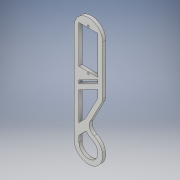
# Autodesk Inventor part: Pata - Brazo
Saved by Autodesk Inventor 2019 (Build 230136000, 136)
## iProperties
Created: 2020-02-12
Part Number: Pata - Brazo
Material: Generic
Document SubType Name: Modeling
Designer: jacqu
Density: 1 g/cm^3
Appearance: Default
Mass: 11.5957 g
Surface Area: 94.6447 cm^2
Volume: 11.5957 cm^3
Author: jacqu
Autodesk Inventor part; units mm, degrees
ref_plane "YZ Plane" through (0, 0, 0) normal (1, 0, 0) x (0, 1, 0)
ref_plane "XZ Plane" through (0, 0, 0) normal (0, 1, 0) x (-1, 0, 0)
ref_plane "XY Plane" through (0, 0, 0) normal (0, 0, 1) x (1, 0, 0)
sketch "Sketch1" plane through (0, 0, 0) normal (0, 0, 1) x (1, 0, 0)
  arc A0 (15, 0) -> (-15, 0) centre (0, 0) ccw
  line L0 (-15, 0) -> (-15, -104)
  line L1 (15, 0) -> (15, -52)
  arc A1 (14.2508, -55.0541) -> (15, -52) centre (8.4, -52) ccw
  arc A2 (-15, -104) -> (-5.2894, -118.0365) centre (0, -104) ccw
  arc A3 (-5.2894, -118.0365) -> (14.9722, -104.9126) centre (0, -104) ccw
  arc A4 (14.9722, -104.9126) -> (5.7487, -90.1453) centre (0, -104) ccw
  arc A5 (1.7228, -79.0541) -> (5.7487, -90.1453) centre (8.8147, -82.7561) ccw
  line L2 (1.7228, -79.0541) -> (14.2508, -55.0541)
  line L3 (-10, 5.5) -> (10, 5.5)
  line L4 (10, 5.5) -> (10, -34.5)
  line L5 (10, -34.5) -> (-10, -34.5)
  line L6 (-10, -34.5) -> (-10, 5.5)
  dimension "d3" = 15
  dimension "d5" = 52
  dimension "d6" = 15
  dimension "d7" = 15
  dimension "d8" = 8
  dimension "d10" = 6.6
  dimension "d11" = 24
  dimension "d17" = 20
  dimension "d18" = 40
  dimension "d19" = 10
  dimension "d20" = 104
  dimension "d30" = 5.5
  constraints: 14 end point, 13 point on circle, 8 tangent, 6 centre point, 3 parallel, 1 coincident, 1 concentric, 1 horizontal, 1 perpendicular, 1 vertical alignment
  measures "d3" radius of A0
  measures "d5" distance of L1.start L1.end
  measures "d6" radius of A2
  measures "d7" radius of A4
  measures "d8" radius of A5
  measures "d10" radius of A1
  measures "d11" vertical distance of L2.start L2.end
  measures "d17" distance of L3.start L3.end
  measures "d18" distance of L3.end L4.end
  measures "d19" distance from line of L6 point (0, 0)
  measures "d20" distance of L0.start L0.end
  measures "d30" distance from line of point (0, 0) L3
extrude "Extrusion1" add sketch "Sketch1" along normal blind 3.3
sketch "Sketch2" plane through (0, 0, 3.3) normal (0, 0, 1) x (1, 0, 0)
  line L0 (-10, 5.5) -> (10, 5.5) projected
  line L1 (10, -34.5) -> (-10, -34.5) projected
  circle A0 centre (0, 7.25) radius 1
  circle A1 centre (0, -36.25) radius 1
  point P0 (0, 0)
  dimension "d31" = 2
  dimension "d32" = 2
  dimension "d34" = 1.75
  dimension "d36" = 1.75
  constraints: 2 centre point, 2 vertical alignment
  measures "d31" diameter of A0
  measures "d32" diameter of A1
  measures "d34" distance from line of L0 A0.centre
  measures "d36" distance from line of L1 A1.centre
extrude "Extrusion2" cut sketch "Sketch2" against normal blind 3.3
sketch "Sketch3" plane through (0, 0, 3.3) normal (0, 0, 1) x (1, 0, 0)
  line L0 (-15, 0) -> (-15, -104) projected
  circle A0 centre (0, 7.25) radius 1 projected
  circle A1 centre (0, -36.25) radius 1 projected
  line L1 (10, 5.5) -> (10, -34.5) projected
  line L2 (10, -34.5) -> (-10, -34.5) projected
  line L3 (-10, -34.5) -> (-10, 5.5) projected
  line L4 (-10, 5.5) -> (10, 5.5) projected
  line L5 (-15, 0) -> (-15, -104) projected
  arc A2 (-15, -104) -> (5.7487, -90.1453) centre (0, -104) ccw projected
  arc A3 (1.7228, -79.0541) -> (5.7487, -90.1453) centre (8.8147, -82.7561) ccw projected
  line L6 (1.7228, -79.0541) -> (14.2508, -55.0541) projected
  arc A4 (14.2508, -55.0541) -> (15, -52) centre (8.4, -52) ccw projected
  line L7 (15, -52) -> (15, 0) projected
  arc A5 (15, 0) -> (-15, 0) centre (0, 0) ccw projected
  line L8 (-10, -86) -> (-10, -56)
  line L9 (10, -45.5723) -> (10, -53.5723)
  line L10 (10, -53.5723) -> (-3.3016, -79.0541)
  line L11 (-3.3016, -79.0541) -> (-10, -86)
  line L12 (1.7228, -79.0541) -> (14.2508, -55.0541) projected
  line L13 (-10, -97.5245) -> (-10, -104)
  arc A6 (-10, -104) -> (3.8325, -94.7635) centre (0, -104) ccw
  arc A7 (-15, -104) -> (5.7487, -90.1453) centre (0, -104) ccw projected
  arc A8 (-2.2846, -89.5242) -> (3.8325, -94.7635) centre (8.8147, -82.7561) ccw
  arc A9 (1.7228, -79.0541) -> (5.7487, -90.1453) centre (8.8147, -82.7561) ccw projected
  line L14 (-2.2846, -89.5242) -> (-10, -97.5245)
  line L15 (-10, -56) -> (10, -45.5723)
  line L16 (-10, -50.3612) -> (10, -39.9336)
  line L17 (10, -39.9336) -> (10, -36.5503)
  line L18 (10, -36.5503) -> (-10, -46.9779)
  line L19 (-10, -46.9779) -> (-10, -50.3612)
  point P0 (14.81, -53.5723)
  dimension "d45" = 5
  dimension "d46" = 5
  dimension "d48" = 8
  dimension "d49" = 18
  dimension "d52" = 5
  dimension "d54" = 3
  dimension "d56" = 30
  dimension "d57" = 8
  constraints: 22 end point, 6 parallel, 5 point on circle, 3 vertical, 3 vertical alignment, 2 centre point, 2 concentric, 2 horizontal alignment, 2 tangent
  measures "d45" distance between parallel lines of L8 L0
  measures "d46" distance between parallel lines of L7 L9
  measures "d48" distance from line of L8.start L14
  measures "d49" vertical distance of L0.end L8.start
  measures "d52" distance between parallel lines of L15 L16
  measures "d54" distance between parallel lines of L16 L18
  measures "d56" distance of L8.start L8.end
  measures "d57" distance of L9.start L9.end
extrude "Extrusion5" cut sketch "Sketch3" against normal blind 10 contours L8 L15 L9 L10 L11 | L14 A8 A6 L13 | L19 L18 L17 L16
equation "\"d3\" = radio_muslo"
equation "\"d6\" = radio_muslo"
equation "\"d7\" = d6"
equation "\"d17\" = base_servo"
equation "\"d18\" = altura_servo"
equation "\"d19\" = 0.5 * base_servo"
equation "\"d20\" = 2 * d5"
equation "\"d22\" = espesor"
equation "\"d31\" = agujero_servo"
equation "\"d32\" = agujero_servo"
equation "\"d34\" = distancia_agujero_servo"
equation "\"d36\" = distancia_agujero_servo"
equation "\"d37\" = espesor"
equation "\"espesor\" = 3.3"
equation "\"radio_muslo\" = 15"
equation "\"base_servo\" = 20"
equation "\"altura_servo\" = 40"
equation "\"agujero_servo\" = 2"
equation "\"distancia_agujero_servo\" = 1.75"
body "Solid1"
